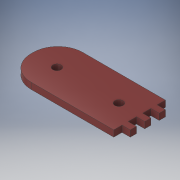
# Autodesk Inventor part: Connection4
Saved by Autodesk Inventor 2019.1 (Build 231200000, 200)
## iProperties
Created: 2018-10-29
Part Number: Connection4
Material: Generic
Document SubType Name: Modeling
Designer: kfortuna
Density: 1 g/cm^3
Appearance: Default
Author: kfortuna
Autodesk Inventor part; units mm, degrees
ref_plane "YZ Plane" through (0, 0, 0) normal (1, 0, 0) x (0, 1, 0)
ref_plane "XZ Plane" through (0, 0, 0) normal (0, 1, 0) x (-1, 0, 0)
ref_plane "XY Plane" through (0, 0, 0) normal (0, 0, 1) x (1, 0, 0)
sketch "Sketch1" plane through (0, 0, 0) normal (0, 1, 0) x (-1, 0, 0)
  line L0 (270.588, 471.9828) -> (250.588, 471.9828)
  line L1 (250.588, 459.4828) -> (270.588, 459.4828)
  line L2 (276.588, 465.4828) -> (276.588, 465.9828)
  arc A0 (276.588, 465.9828) -> (270.588, 471.9828) centre (270.588, 465.9828) ccw
  arc A1 (270.588, 459.4828) -> (276.588, 465.4828) centre (270.588, 465.4828) ccw
  circle A2 centre (270.588, 465.7328) radius 1
  line L3 (250.588, 459.4828) -> (250.588, 461.4828)
  line L4 (250.588, 461.4828) -> (248.588, 461.4828)
  line L5 (248.588, 462.9828) -> (250.588, 462.9828)
  line L6 (250.588, 462.9828) -> (250.588, 464.9828)
  line L7 (250.588, 464.9828) -> (248.588, 464.9828)
  line L8 (248.588, 466.4828) -> (250.588, 466.4828)
  line L9 (250.588, 466.4828) -> (250.588, 468.4828)
  line L10 (250.588, 468.4828) -> (248.588, 468.4828)
  line L11 (248.588, 462.9828) -> (248.588, 461.4828)
  line L12 (248.588, 469.9828) -> (248.588, 468.4828)
  line L13 (248.588, 466.4828) -> (248.588, 464.9828)
  line L14 (248.588, 469.9828) -> (250.588, 469.9828)
  line L15 (250.588, 469.9828) -> (250.588, 471.9828)
  point P0 (0, 0)
  point P1 (276.588, 471.9828)
  point P2 (276.588, 459.4828)
  dimension "d2" = 6
  dimension "d5" = 2
  dimension "d15" = 0
  dimension "d26" = 2
  dimension "d27" = 2
  dimension "d28" = 2
  dimension "d29" = 2
  dimension "d30" = 2
  dimension "d31" = 2
  dimension "d32" = 1.5
  dimension "d33" = 1.5
  dimension "d34" = 2
  dimension "d35" = 1.5
  dimension "d36" = 2
  dimension "d39" = 20
  constraints: 32 end point, 8 perpendicular, 8 point on line, 6 parallel, 4 point on circle, 4 tangent, 3 centre point, 2 horizontal, 1 equal radius, 1 vertical
  measures "d2" radius of A0
  measures "d5" diameter of A2
  measures "d15" horizontal distance of A0.centre A2.centre
  measures "d26" distance of L3.end L4.end
  measures "d27" distance of L6.end L7.end
  measures "d28" distance of L9.end L10.end
  measures "d29" distance of L1.start L3.end
  measures "d30" distance of L5.end L6.end
  measures "d31" distance between parallel lines of L8 L10
  measures "d32" distance of L5.start L4.end
  measures "d33" distance of L8.start L7.end
  measures "d34" distance of L12.start L14.end
  measures "d35" distance of L12.start L10.end
  measures "d36" distance of L14.end L0.end
  measures "d39" distance of L1.start L1.end
extrude "Extrusion7" add sketch "Sketch1" along normal blind 1.524
sketch "Sketch2" plane through (0, 1.524, 0) normal (0, 1, 0) x (1, 0, 0)
  circle A0 centre (-255.588, -465.7328) radius 1
  line L0 (-250.588, -459.4828) -> (-270.588, -459.4828) projected
  line L1 (-250.588, -461.4828) -> (-250.588, -459.4828) projected
  circle A1 centre (-270.588, -465.7328) radius 1 projected
  line L2 (-270.588, -471.9828) -> (-250.588, -471.9828) projected
  point P0 (0, 0)
  dimension "d40" = 2
  dimension "d43" = 15
  dimension "d44" = 6.25
  constraints: 1 centre point
  measures "d40" diameter of A0
  measures "d43" distance of A1.centre A0.centre
  measures "d44" distance from line of L2 A0.centre
extrude "Extrusion8" cut sketch "Sketch2" against normal blind 10 contours A0
body "Solid5"
